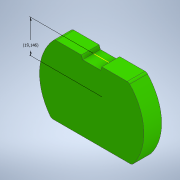
# Autodesk Inventor part: vydacha_disk
Saved by Autodesk Inventor 2020 (Build 240168000, 168)
## iProperties
Created: 2022-07-26
Part Number: vydacha_disk
Material: Типовые
Document SubType Name: Modeling
Designer: akapu
Density: 1 g/cm^3
Appearance: По умолчанию
Author: akapu
Autodesk Inventor part; units mm, degrees
ref_plane "YZ Plane" through (0, 0, 0) normal (1, 0, 0) x (0, 1, 0)
ref_plane "XZ Plane" through (0, 0, 0) normal (0, 1, 0) x (-1, 0, 0)
ref_plane "XY Plane" through (0, 0, 0) normal (0, 0, 1) x (1, 0, 0)
sketch "Эскиз5" plane through (0, 0, 0) normal (0, 0, 1) x (1, 0, 0)
  circle A0 centre (0, 0) radius 30
  line L0 (0, 30) -> (-5.2, 30)
  line L1 (-5.2, 30) -> (-5.2, 29.5459)
  line L2 (-5.2, 29.5459) -> (-5.2, 19.1459)
  line L3 (-5.2, 19.1459) -> (5.2, 19.1459)
  line L4 (5.2, 19.1459) -> (5.2, 29.5459)
  dimension "d17" = 60
  dimension "d18" = 5.2
  dimension "d19" = 10.4
  dimension "d20" = 10.4
  constraints: 10 end point, 3 point on circle, 2 perpendicular, 1 centre point, 1 coincident, 1 horizontal, 1 tangent, 1 vertical
  measures "d17" diameter of A0
  measures "d18" distance of L0.start L0.end
  measures "d19" distance of L1.end L2.end
  measures "d20" distance of L2.end L3.end
extrude "Выдавливание3" add sketch "Эскиз5" along normal blind 10.2 contours A0 L2 L3 L4 picked at (-1.0099, 2.8151)
sketch "Эскиз7" plane through (0, 0, 10.2) normal (0, 0, 1) x (1, 0, 0)
  line L0 (5.2, 19.1459) -> (-5.2, 19.1459) projected
  line L1 (-5.2, 19.1459) -> (-5.2, 21.1459)
  line L2 (-5.2, 21.1459) -> (21.2803, 21.1459)
  arc A0 (-5.2, 29.5459) -> (5.2, 29.5459) centre (0, 0) ccw projected
  line L3 (-5.2, 21.1459) -> (-21.3192, 21.1459)
  line L4 (-5.2, 19.1459) -> (-5.2, 29.5459) projected
  circle A1 centre (0, 0) radius 30
  point P0 (-21.2803, 21.1459)
  point P1 (5.2, 29.5459)
  dimension "d26" = 2
  constraints: 6 end point, 1 coincident, 1 perpendicular, 1 point on circle, 1 point on line, 1 vertical, 3 other
  measures "d26" distance of L0.end L1.end
extrude "Выдавливание5" cut sketch "Эскиз7" against normal blind 11 contours L4 A1 A0 L2 | L3 A0 L4
sketch "Эскиз8" plane through (0, 0, 10.2) normal (0, 0, 1) x (1, 0, 0)
  line L0 (-5.2, 21.1459) -> (-21.2803, 21.1459) projected
  line L1 (-5.2, 21.1459) -> (-5.9, 21.1459)
  line L2 (-5.2, 19.1459) -> (-5.2, 21.1459) projected
  line L3 (-5.9, 21.1459) -> (-5.2, 19.1459)
  line L4 (5.2, 21.1459) -> (5.2, 19.1459) projected
  line L5 (-5.2, 19.1459) -> (5.2, 19.1459)
  line L6 (5.2, 19.1459) -> (5.2, 21.1459)
  line L7 (5.2, 21.1459) -> (5.9, 21.1459)
  line L8 (21.2803, 21.1459) -> (5.2, 21.1459) projected
  line L9 (5.9, 21.1459) -> (5.2, 19.1459)
  point P0 (0, 0)
  dimension "d29" = 0.7
  dimension "d30" = 0.7
  constraints: 12 end point, 2 point on line, 1 collinear, 1 perpendicular
  measures "d29" distance of L0.start L1.end
  measures "d30" distance of L4.start L7.end
extrude "Выдавливание6" cut sketch "Эскиз8" against normal blind 11
sketch "Эскиз9" plane through (0, 0, 10.2) normal (0, 0, 1) x (1, 0, 0)
  line L0 (0, 0) -> (0, -19)
  line L1 (0, -19) -> (23.2164, -19)
  arc A0 (-21.2803, 21.1459) -> (21.2803, 21.1459) centre (0, 0) ccw projected
  line L2 (0, -19) -> (-23.2164, -19)
  circle A1 centre (0, 0) radius 30
  dimension "d33" = 19
  constraints: 6 end point, 2 point on circle, 1 centre point, 1 coincident, 1 concentric, 1 horizontal, 1 perpendicular, 1 vertical
  measures "d33" distance of L0.start L0.end
extrude "Выдавливание7" cut sketch "Эскиз9" against normal blind 11 contours L1 A0 L2
fillet "Сопряжение1" radius 2 2 edges at (23.2164, -19, 5.1) (21.2803, 21.1459, 5.1)
sketch "Эскиз10" plane through (0, 0, 0) normal (0, 0, -1) x (-1, 0, 0)
  circle A0 centre (0, 0) radius 6.5
  circle A1 centre (0, 0) radius 5
  line L0 (0, 0) -> (19, 0)
  line L1 (19, 0) -> (-19, 0)
  line L2 (-19, 0) -> (-16.5, 0)
  line L3 (19, 0) -> (16.5, 0)
  circle A2 centre (-16.5, 0) radius 2.75
  circle A3 centre (16.5, 0) radius 2.75
  line L4 (0, 5) -> (-16.5, 2.75)
  line L5 (0, 5) -> (16.5, 2.75)
  line L6 (16.5, -2.75) -> (0, -5)
  line L7 (0, -5) -> (-16.5, -2.75)
  point P0 (-4.8387, -4.3402)
  point P1 (4.8387, -4.3402)
  point P2 (4.8387, 4.3402)
  point P3 (-4.8387, 4.3402)
  dimension "d39" = 13
  dimension "d40" = 10
  dimension "d41" = 19
  dimension "d42" = 38
  dimension "d43" = 2.5
  dimension "d44" = 2.5
  dimension "d45" = 5.5
  dimension "d46" = 5.5
  constraints: 16 end point, 6 point on circle, 4 centre point, 3 coincident, 3 point on line, 2 parallel, 1 horizontal
  measures "d39" diameter of A0
  measures "d40" diameter of A1
  measures "d41" distance of L0.start L0.end
  measures "d42" distance of L0.end L1.end
  measures "d43" distance of L1.end L2.end
  measures "d44" distance of L0.end L3.end
  measures "d45" diameter of A2
  measures "d46" diameter of A3
extrude "Выдавливание8" cut sketch "Эскиз10" against normal blind 4
sketch "Эскиз12" plane through (0, 0, 0) normal (0, 0, -1) x (-1, 0, 0)
  point P0 (0, 0)
sketch "Эскиз13" plane through (0, 0, 4) normal (0, 0, -1) x (-1, 0, 0)
  line L0 (-5.2, 19.1459) -> (5.2, 19.1459) projected
  point P0 (0, 0)
  dimension "d49" = 19.1459
  measures "d49" distance from line of point (0, 0) L0
